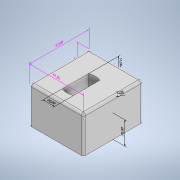
# Autodesk Inventor part: PVC_Camera_Adaptator
Saved by Autodesk Inventor 2020.3 (Build 243373000, 373)
## iProperties
Created: 2021-02-23
Part Number: PVC_Camera_Adaptator
Material: Generic
Document SubType Name: Modeling
Designer: super
Density: 1 g/cm^3
Appearance: Default
Author: super
Autodesk Inventor part; units mm, degrees
ref_plane "YZ Plane" through (0, 0, 0) normal (1, 0, 0) x (0, 1, 0)
ref_plane "XZ Plane" through (0, 0, 0) normal (0, 1, 0) x (-1, 0, 0)
ref_plane "XY Plane" through (0, 0, 0) normal (0, 0, 1) x (1, 0, 0)
sketch "Sketch1" plane through (0, 0, 0) normal (0, 1, 0) x (-1, 0, 0)
  line L0 (0, 0) -> (-47, 0)
  line L1 (-47, 0) -> (-47, -52)
  line L2 (-47, -52) -> (0, -52)
  line L3 (0, -52) -> (0, 0)
  dimension "d0" = 47
  dimension "d1" = 52
  constraints: 8 end point, 2 parallel, 1 horizontal, 1 perpendicular
  measures "d0" distance of L2.end L1.end
  measures "d1" distance of L1.end L0.end
extrude "Extrusion1" add sketch "Sketch1" along normal blind 32
sketch "Sketch2" plane through (0, 32, 0) normal (0, 1, 0) x (1, 0, 0)
  line L0 (0, 0) -> (47, 0) projected
  line L1 (0, 52) -> (0, 0) projected
  line L2 (47, 0) -> (47, 52) projected
  line L3 (28.5, 21.5) -> (28.5, 34)
  line L4 (28.5, 34) -> (18.5, 34)
  line L5 (18.5, 34) -> (18.5, 9)
  line L6 (18.5, 9) -> (28.5, 9)
  line L7 (28.5, 9) -> (28.5, 21.5)
  circle A0 centre (23.5, 21.5) radius 12.5
  point P0 (28.5, 10.0436)
  point P1 (28.5, 32.9564)
  point P2 (18.5, 32.9564)
  point P3 (18.5, 10.0436)
  dimension "d7" = 12.5
  dimension "d8" = 10
  dimension "d9" = 25
  dimension "d10" = 25
  constraints: 10 end point, 4 perpendicular, 1 centre point, 1 point on line
  measures "d7" distance of L3.start L3.end
  measures "d8" distance of L3.end L4.end
  measures "d9" distance of L4.end L5.end
  measures "d10" diameter of A0
extrude "Extrusion2" cut sketch "Sketch2" against normal blind 11 contours L7 A0 L5 L3
sketch "Sketch3" plane through (0, 0, 0) normal (0, -1, 0) x (1, 0, 0)
  line L0 (0, -52) -> (0, 0) projected
  line L1 (47, 0) -> (47, -52) projected
  circle A0 centre (23.5, -26) radius 13.5
  circle A1 centre (23.5, -26) radius 10.5
  dimension "d15" = 27
  dimension "d16" = 21
  constraints: 2 centre point, 1 coincident
  measures "d15" diameter of A0
  measures "d16" diameter of A1
extrude "Extrusion3" cut sketch "Sketch3" against normal blind 20
fillet "Fillet1" radius 2 8 edges at (23.5, 32, 0) (47, 32, -26) (23.5, 32, -52) (47, 16, -52) (47, 16, 0) (0, 16, -52) (0, 32, -26) (0, 16, 0)
body "Solid1"
